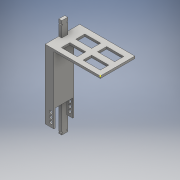
# Autodesk Inventor part: GrapperRight
Saved by Autodesk Inventor 2016 (Build 200138000, 138)
## iProperties
Created: 2016-03-30
Part Number: GrapperRight
Material: Generic
Document SubType Name: Modeling
Designer: mkepler
Density: 1 g/cm^3
Appearance: Default
Mass: 12.3787 g
Surface Area: 108.063 cm^2
Volume: 12.3787 cm^3
Author: mkepler
Autodesk Inventor part; units mm, degrees
ref_plane "YZ Plane" through (0, 0, 0) normal (1, 0, 0) x (0, 1, 0)
ref_plane "XZ Plane" through (0, 0, 0) normal (0, 1, 0) x (-1, 0, 0)
ref_plane "XY Plane" through (0, 0, 0) normal (0, 0, 1) x (1, 0, 0)
sketch "Sketch3" plane through (0, 0, 0) normal (0, 1, 0) x (-1, 0, 0)
  line L0 (0, 0) -> (70, 0)
  line L1 (70, 0) -> (70, -70)
  line L2 (70, -70) -> (70, -94)
  line L3 (70, -94) -> (64, -94)
  line L4 (64, -94) -> (64, -70)
  line L5 (64, -3) -> (0, -3)
  line L6 (0, -3) -> (0, 0)
  line L7 (64, -70) -> (67, -70)
  line L8 (67, -70) -> (67, -3)
  line L9 (67, -3) -> (64, -3)
  circle A0 centre (67, -82) radius 2.125
  circle A1 centre (67, -76) radius 2.125
  circle A2 centre (67, -88) radius 2.125
  dimension "d26" = 70
  dimension "d27" = 70
  dimension "d29" = 6
  dimension "d55" = 4.25
  dimension "d56" = 4.25
  dimension "d57" = 4.25
  dimension "d59" = 6
  dimension "d60" = 6
  dimension "d61" = 6
  constraints: 20 end point, 6 perpendicular, 3 centre point, 2 horizontal, 2 point on line, 1 parallel
  measures "d26" distance of L0.start L0.end
  measures "d27" distance of L0.end L1.end
  measures "d29" distance of L2.end L3.end
  measures "d55" diameter of A0
  measures "d56" diameter of A1
  measures "d57" diameter of A2
  measures "d59" distance of A0.centre A2.centre
  measures "d60" distance from line of L7 A1.centre
  measures "d61" distance of A0.centre A1.centre
extrude "Extrusion2" add sketch "Sketch3" along normal blind 27 contours L0 L1 L2 L3 L4 L7 L8 L9 L5 L6 | A0 | A1 | A2
sketch "Sketch4" plane through (0, 27, 0) normal (0, 1, 0) x (1, 0, 0)
  line L0 (-70, 0) -> (0, 0) projected
  line L1 (0, 0) -> (0, 3) projected
  line L2 (-70, 0) -> (0, 0)
  line L3 (0, 0) -> (0, 3)
  line L4 (0, 3) -> (-70, 3)
  line L5 (-70, 3) -> (-70, 0)
  constraints: 8 end point, 2 parallel, 1 horizontal, 1 perpendicular
extrude "Extrusion3" add sketch "Sketch4" along normal blind 20
sketch "Sketch5" plane through (-70, 0, -94) normal (-1, 0, 0) x (0, 0, 1)
  line L0 (-0.1204, 1.5) -> (23.8796, 1.5)
  line L1 (23.8796, 1.5) -> (23.8796, 25.5)
  line L2 (23.8796, 25.5) -> (-0.1204, 25.5)
  line L3 (-0.1204, 25.5) -> (-0.1204, 1.5)
  line L4 (94, 0) -> (0, 0) projected
  dimension "d36" = 24
  dimension "d37" = 24
  dimension "d38" = 1.5
  constraints: 8 end point, 2 parallel, 1 horizontal, 1 perpendicular
  measures "d36" distance of L2.end L1.end
  measures "d37" distance of L1.end L0.end
  measures "d38" distance between parallel lines of L0 L4
extrude "Extrusion4" cut sketch "Sketch5" against normal blind 10
sketch "Sketch9" plane through (0, 0, -3) normal (0, 0, -1) x (-1, 0, 0)
  line L0 (7, 7) -> (60, 7)
  line L1 (60, 7) -> (60, 39)
  line L2 (60, 39) -> (7, 39)
  line L3 (7, 39) -> (7, 7)
  line L4 (0, 0) -> (0, 47) projected
  line L5 (67, 0) -> (0, 0) projected
  dimension "d45" = 53
  dimension "d46" = 32
  dimension "d47" = 7
  dimension "d48" = 7
  constraints: 8 end point, 2 parallel, 1 horizontal, 1 perpendicular
  measures "d45" distance of L2.end L1.end
  measures "d46" distance of L1.end L0.end
  measures "d47" distance between parallel lines of L4 L3
  measures "d48" distance between parallel lines of L5 L0
extrude "Extrusion5" cut sketch "Sketch9" against normal blind 10
sketch "Sketch10" plane through (-70, 0, 0) normal (0, 0, 1) x (1, 0, 0)
  line L0 (10, 39) -> (10, 7) projected
  line L1 (63, 7) -> (63, 39) projected
  line L2 (63, 26.6385) -> (63, 18.6385)
  line L3 (10, 18.6385) -> (10, 26.6385)
  line L4 (63, 39) -> (10, 39) projected
  line L5 (10, 7) -> (63, 7) projected
  line L6 (31.6097, 39) -> (39.6097, 39)
  line L7 (39.6097, 39) -> (39.6097, 7)
  line L8 (39.6097, 7) -> (31.6097, 7)
  line L9 (31.6097, 7) -> (31.6097, 18.6385)
  line L10 (31.6097, 26.6385) -> (31.6097, 39)
  line L11 (10, 26.6385) -> (31.6097, 26.6385)
  line L12 (39.6097, 26.6385) -> (63, 26.6385)
  line L13 (63, 18.6385) -> (39.6097, 18.6385)
  line L14 (31.6097, 18.6385) -> (10, 18.6385)
  point P0 (70, 0)
  dimension "d51" = 8
  dimension "d52" = 8
  constraints: 22 end point, 8 parallel, 6 point on line, 3 horizontal, 3 perpendicular
  measures "d51" distance of L2.start L2.end
  measures "d52" distance of L7.end L8.end
extrude "Extrusion6" add sketch "Sketch10" against normal blind 3 contours L11 L10 L4 L7 L5 L9 L14 L0 | L12 L1 L13 L7
sketch "Sketch11" plane through (0, 0, 0) normal (0, -1, 0) x (1, 0, 0)
  point P0 (0, 0)
sketch "Sketch12" plane through (0, 0, 0) normal (0, -1, 0) x (1, 0, 0)
  circle A0 centre (-67, -82) radius 2.125
  circle A1 centre (-67, -76) radius 2.125
  circle A2 centre (-67, -88) radius 2.125
  line L0 (-64, -70) -> (-67, -70) projected
  point P0 (0, 0)
  dimension "d62" = 4.25
  dimension "d63" = 4.25
  dimension "d64" = 4.25
  dimension "d65" = 6
  dimension "d66" = 6
  dimension "d67" = 6
  constraints: 3 centre point
  measures "d62" diameter of A0
  measures "d63" diameter of A1
  measures "d64" diameter of A2
  measures "d65" distance from line of L0 A1.centre
  measures "d66" distance of A0.centre A2.centre
  measures "d67" distance of A1.centre A0.centre
hole "Hole2" at (-67, 0, -88) at (-67, 0, -82) at (-67, 0, -76) direction (0, 1, 0) diameter 4.25 end through all
sketch "Sketch15" plane through (-67, 0, -3) normal (1, 0, 0) x (0, 0, -1)
  line L0 (67, 0) -> (67, 27) projected
  line L1 (67, 0) -> (0, 0) projected
  line L2 (67, 0) -> (0, 0)
  line L3 (0, 0) -> (0, 27) projected
  line L4 (0, 0) -> (0, 27)
  line L5 (0, 27) -> (67, 27)
  line L6 (67.1204, 25.5) -> (67.1204, 1.5) projected
  line L7 (67.1204, 25.5) -> (67.1204, 1.5)
  line L8 (67.1204, 1.5) -> (67, 0)
  line L9 (67, 27) -> (67, 0)
  point P0 (-3, 0)
  constraints: 12 end point, 2 collinear, 1 parallel, 1 perpendicular, 1 vertical
extrude "Extrusion7" add sketch "Sketch15" along normal blind 3
sketch "Sketch18" plane through (-64, 0, -3) normal (1, 0, 0) x (0, 0, -1)
  line L0 (0, 0) -> (0, 27) projected
  line L1 (0, 27) -> (0, 0)
  line L2 (91, 0) -> (0, 0) projected
  line L3 (0, 0) -> (91, 0)
  line L4 (91, 0) -> (91, 1.5) projected
  line L5 (91, 0) -> (91, 1.5)
  line L6 (67.1204, 1.5) -> (67.1204, 25.5) projected
  line L7 (91, 1.5) -> (67.1204, 1.5)
  line L8 (67.1204, 25.5) -> (67.1204, 1.5) projected
  line L9 (67.1204, 1.5) -> (67.1204, 25.5)
  line L10 (67.1204, 25.5) -> (91, 25.5) projected
  line L11 (67.1204, 25.5) -> (91, 25.5)
  line L12 (91, 27) -> (0, 27) projected
  line L13 (91, 25.5) -> (91, 27)
  line L14 (91, 27) -> (0, 27)
  point P0 (-3, 0)
  constraints: 16 end point, 5 collinear, 3 perpendicular
extrude "Extrusion8" add sketch "Sketch18" along normal blind 1
sketch "Sketch19" plane through (-70, 0, -94) normal (-1, 0, 0) x (0, 0, 1)
  line L0 (94, 47) -> (94, 0)
  line L1 (91, 0) -> (0, 0) projected
  line L2 (94, 0) -> (0, 0)
  line L3 (0, 0) -> (0, 1.5) projected
  line L4 (0, 0) -> (0, 1.5)
  line L5 (23.8796, 25.5) -> (23.8796, 1.5) projected
  line L6 (0, 1.5) -> (23.8796, 1.5)
  line L7 (23.8796, 1.5) -> (23.8796, 25.5)
  line L8 (23.8796, 25.5) -> (0, 25.5) projected
  line L9 (23.8796, 25.5) -> (0, 25.5)
  line L10 (0, 27) -> (91, 27) projected
  line L11 (0, 25.5) -> (0, 27)
  line L12 (0, 27) -> (91, 27)
  line L13 (91, 27) -> (91, 47) projected
  line L14 (91, 27) -> (91, 47)
  line L15 (91, 47) -> (94, 47) projected
  line L16 (91, 47) -> (94, 47)
  constraints: 20 end point, 5 perpendicular, 3 collinear, 2 vertical, 1 point on line
extrude "Extrusion9" add sketch "Sketch19" along normal blind 1
sketch "Sketch20" plane through (-71, 0, -94) normal (-1, 0, 0) x (0, 0, 1)
  line L0 (94, 26.6385) -> (94, 39) projected
  line L1 (94, 26.6385) -> (114.5, 26.6385)
  line L2 (114.5, 26.6385) -> (114.5, 18.6385)
  line L3 (94, 18.6385) -> (94, 7) projected
  line L4 (114.5, 18.6385) -> (94, 18.6385)
  line L5 (94, 18.6385) -> (0, 18.6385)
  line L6 (0, 18.6385) -> (-20.5, 18.6385)
  line L7 (-20.5, 18.6385) -> (-20.5, 26.6385)
  line L8 (-20.5, 26.6385) -> (94, 26.6385)
  point P0 (94, 0)
  dimension "d81" = 20.5
  dimension "d82" = 94
  dimension "d83" = 20.5
  dimension "d84" = 180
  constraints: 14 end point, 4 perpendicular, 1 collinear, 1 horizontal, 1 point on line
  measures "d81" distance of L0.start L1.end
  measures "d82" distance of L3.start L5.end
  measures "d83" distance of L5.end L6.end
  measures "d84" angle of L6 L5
extrude "Extrusion10" add sketch "Sketch20" along normal blind 2
sketch "Sketch21" plane through (-71, 0, -94) normal (-1, 0, 0) x (0, 0, 1)
  line L0 (94, 18.6385) -> (94, 7) projected
  line L1 (94, 0) -> (94, 18.6385)
  line L2 (94, 18.6385) -> (23.8796, 18.6385) projected
  line L3 (94, 18.6385) -> (23.8796, 18.6385)
  line L4 (23.8796, 1.5) -> (23.8796, 25.5) projected
  line L5 (23.8796, 18.6385) -> (23.8796, 1.5)
  line L6 (91, 0) -> (0, 0) projected
  line L7 (23.8796, 1.5) -> (0, 1.5) projected
  line L8 (23.8796, 1.5) -> (0, 1.5)
  line L9 (0, 1.5) -> (0, 0) projected
  line L10 (0, 1.5) -> (0, 0)
  line L11 (0, 0) -> (94, 0)
  constraints: 12 end point, 3 perpendicular, 2 collinear, 1 horizontal
extrude "Extrusion11" add sketch "Sketch21" along normal blind 2
sketch "Sketch22" plane through (-71, 0, -94) normal (-1, 0, 0) x (0, 0, 1)
  line L0 (91, 27) -> (0, 27) projected
  line L1 (0, 27) -> (0, 26.6385) projected
  line L2 (0, 27) -> (0, 26.6385)
  line L3 (0, 25.5) -> (0, 27) projected
  line L4 (94, 26.6385) -> (94, 47) projected
  line L5 (0, 26.6385) -> (94, 26.6385)
  line L6 (94, 26.6385) -> (94, 47)
  line L7 (94, 47) -> (91, 47) projected
  line L8 (94, 47) -> (91, 47)
  line L9 (91, 47) -> (91, 27) projected
  line L10 (91, 47) -> (91, 27)
  line L11 (91, 27) -> (0, 27)
  point P0 (94, 0)
  constraints: 12 end point, 5 perpendicular, 1 collinear
extrude "Extrusion12" add sketch "Sketch22" along normal blind 2
sketch "Sketch23" plane through (-73, 0, -94) normal (-1, 0, 0) x (0, 0, 1)
  line L0 (94, 0) -> (94, 47) projected
  line L1 (94, 18.6385) -> (94, 26.6385) projected
  line L2 (94, 0) -> (94, 18.6385)
  line L3 (114.5, 18.6385) -> (114.5, 26.6385) projected
  line L4 (94, 18.6385) -> (114.5, 18.6385)
  line L5 (114.5, 18.6385) -> (114.5, 26.6385)
  line L6 (114.5, 26.6385) -> (94, 26.6385)
  line L7 (94, 26.6385) -> (94, 47)
  line L8 (94, 47) -> (91, 47) projected
  line L9 (94, 47) -> (91, 47)
  line L10 (0, 27) -> (91, 27) projected
  line L11 (91, 47) -> (91, 27)
  line L12 (91, 26.6385) -> (91, 39) projected
  line L13 (91, 27) -> (0, 27)
  line L14 (0, 26.6385) -> (-20.5, 26.6385) projected
  line L15 (0, 27) -> (0, 26.6385)
  line L16 (0, 25.5) -> (0, 27) projected
  line L17 (0, 26.6385) -> (-20.5, 26.6385)
  line L18 (-20.5, 26.6385) -> (-20.5, 18.6385) projected
  line L19 (-20.5, 26.6385) -> (-20.5, 18.6385)
  line L20 (-20.5, 18.6385) -> (23.8796, 18.6385) projected
  line L21 (-20.5, 18.6385) -> (23.8796, 18.6385)
  line L22 (23.8796, 18.6385) -> (23.8796, 1.5) projected
  line L23 (23.8796, 18.6385) -> (23.8796, 1.5)
  line L24 (0, 1.5) -> (0, 0) projected
  line L25 (23.8796, 1.5) -> (0, 1.5)
  line L26 (0, 1.5) -> (0, 0)
  line L27 (0, 0) -> (94, 0) projected
  line L28 (0, 0) -> (94, 0)
  constraints: 32 end point, 9 collinear, 6 perpendicular, 1 horizontal
extrude "Extrusion13" add sketch "Sketch23" along normal blind 2
sketch "Sketch24" plane through (-75, 0, -94) normal (-1, 0, 0) x (0, 0, 1)
  line L0 (-17.5, 26.6385) -> (-17.5, 25.1385)
  line L1 (-17.5, 25.1385) -> (-18.5, 25.1385)
  line L2 (-18.5, 25.1385) -> (-18.5, 26.6385)
  line L3 (-17.5, 26.6385) -> (-17.5, 25.1385)
  line L4 (-17.5, 26.6385) -> (-18.5, 26.6385)
  line L5 (-20.5, 26.6385) -> (0, 26.6385) projected
  line L6 (-20.5, 18.6385) -> (-20.5, 26.6385) projected
  line L7 (-20.5, 22.6385) -> (-27.0892, 22.6385)
  line L8 (-17.5, 18.6385) -> (-17.5, 20.1385)
  line L9 (-17.5, 20.1385) -> (-18.5, 20.1385)
  line L10 (-18.5, 20.1385) -> (-18.5, 18.6385)
  line L11 (-17.5, 18.6385) -> (-18.5, 18.6385)
  line L12 (91, 0) -> (0, 0) projected
  line L13 (45.5, 0) -> (45.5, 18.6385)
  line L14 (108.5, 26.6385) -> (108.5, 25.1385)
  line L15 (108.5, 25.1385) -> (109.5, 25.1385)
  line L16 (109.5, 25.1385) -> (109.5, 26.6385)
  line L17 (108.5, 18.6385) -> (108.5, 20.1385)
  line L18 (108.5, 20.1385) -> (109.5, 20.1385)
  line L19 (109.5, 20.1385) -> (109.5, 18.6385)
  line L20 (108.5, 18.6385) -> (109.5, 18.6385)
  line L21 (108.5, 26.6385) -> (109.5, 26.6385)
  line L22 (94, 26.6385) -> (114.5, 26.6385) projected
  point P0 (94, 0)
  dimension "d93" = 17.5
  dimension "d94" = 1.5
  dimension "d95" = 1
  constraints: 38 end point, 12 symmetric about line, 2 collinear, 2 midpoint, 2 perpendicular, 1 horizontal, 1 parallel, 1 vertical
  measures "d93" distance of L5.end L0.start
  measures "d94" distance of L0.start L0.end
  measures "d95" distance of L0.end L1.end
extrude "Extrusion14" cut sketch "Sketch24" against normal through all
body "Solid2"
